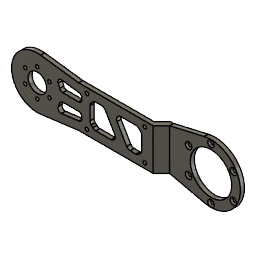
maker arm cnc装配 (Autodesk Fusion 360 archive; units mm, degrees)
design "L2输出侧臂"
part number: 2026-08-07-18-40-20-712
Autodesk Fusion 360 part; units mm, degrees
note: some values were not read from the file. Set by a fixed rule: the direction of a hole.
(part 1 of 4)
sketch "草图1" plane through (0, 0, 0) normal (0, 0, 1) x (1, 0, 0)
  line L0 (0, -20) -> (160, -20)
  arc A0 (160, -20) -> (160, 20) centre (160, 0) ccw
  line L1 (160, 20) -> (0, 20)
  arc A1 (0, 20) -> (0, -20) centre (0, 0) ccw
  line L2 (0, 0) -> (160, 0) construction
  line L3 (-10.3229, -9.3593) -> (-6.3955, -5.4319)
  arc A2 (-2.9439, 13.6195) -> (-5.8655, 15.1009) centre (-5.0689, 13.0501) ccw
  circle A3 centre (0, -13.5) radius 1.6
  arc A4 (16.0105, 2.4708) -> (13.2668, 4.2603) centre (13.8362, 2.1352) ccw
  circle A5 centre (-11.6913, 6.75) radius 1.6
  arc A6 (-5.8655, 15.1009) -> (-10.145, 12.6301) centre (0, 0) ccw
  line L4 (-1.5064, -8.2546) -> (-2.9439, -13.6195)
  circle A7 centre (-11.6913, -6.75) radius 1.6
  line L5 (7.9019, 2.8227) -> (13.2668, 4.2603)
  arc A8 (-2.6915, 5.6961) -> (-1.5064, 8.2547) centre (-3.6314, 7.6852) ccw
  circle A9 centre (6.115, -10.5915) radius 1.7
  circle A10 centre (6.115, 10.5915) radius 1.7
  circle A11 centre (11.6913, -6.75) radius 1.6
  circle A12 centre (11.6913, 6.75) radius 1.6
  arc A13 (-10.145, 12.6301) -> (-10.3229, 9.3593) centre (-8.7673, 10.9149) ccw
  arc A14 (-10.145, -12.6301) -> (-5.8655, -15.1009) centre (0, 0) ccw
  arc A15 (-2.6915, 5.6961) -> (-3.5872, 5.179) centre (0, 0) ccw
  arc A16 (13.2668, -4.2603) -> (16.0105, -2.4708) centre (13.8362, -2.1352) ccw
  arc A17 (6.2787, -0.5171) -> (7.9019, -2.8228) centre (8.4713, -0.6977) ccw
  circle A18 centre (0, 0) radius 18
  arc A19 (-1.5064, -8.2546) -> (-2.6915, -5.6961) centre (-3.6314, -7.6852) ccw
  circle A20 centre (-12.23, 0) radius 1.7
  line L6 (-6.3955, 5.4319) -> (-10.3229, 9.3593)
  circle A21 centre (0, 13.5) radius 1.6
  arc A22 (7.9019, 2.8227) -> (6.2787, 0.5171) centre (8.4713, 0.6977) ccw
  line L7 (-2.9439, 13.6195) -> (-1.5064, 8.2547)
  arc A23 (-5.8655, -15.1009) -> (-2.9439, -13.6195) centre (-5.0689, -13.0501) ccw
  arc A24 (6.2787, -0.5171) -> (6.2787, 0.5171) centre (0, 0) ccw
  arc A25 (-10.3229, -9.3593) -> (-10.145, -12.6301) centre (-8.7673, -10.9149) ccw
  arc A26 (16.0105, -2.4708) -> (16.0105, 2.4708) centre (0, 0) ccw
  arc A27 (-6.3955, 5.4319) -> (-3.5872, 5.179) centre (-4.8399, 6.9875) ccw
  line L8 (13.2668, -4.2603) -> (7.9019, -2.8228)
  circle A28 centre (0, 0) radius 4.75
  arc A29 (-3.5872, -5.179) -> (-2.6915, -5.6961) centre (0, 0) ccw
  arc A30 (-3.5872, -5.179) -> (-6.3955, -5.4319) centre (-4.8399, -6.9875) ccw
  circle A31 centre (160, 0) radius 28.5
  line L9 (153.5772, 27.7668) -> (120, 20)
  line L10 (120, -20) -> (153.5772, -27.7668)
  circle A32 centre (160, 0) radius 20
  circle A33 centre (160, 0) radius 25 construction
  circle A34 centre (160, 25) radius 1.65
  circle A35 centre (138.3494, 12.5) radius 1.65
  circle A36 centre (138.3494, -12.5) radius 1.65
  circle A37 centre (160, -25) radius 1.65
  circle A38 centre (181.6506, -12.5) radius 1.65
  circle A39 centre (181.6506, 12.5) radius 1.65
  circle A40 centre (0, 0) radius 25
  line L11 (3.2298, 24.7905) -> (40, 20)
  line L12 (3.2298, -24.7905) -> (40, -20)
  line L13 (160, 0) -> (160, 50)
  line L14 (160, 0) -> (160, 25)
  point P0 (0, 0)
  dimension "d1" = 20
  dimension "d2" = 160
  dimension "d3" = 36
  dimension "d4" = 3.2
  dimension "d5" = 57
  dimension "d6" = 40
  dimension "d7" = 40
  dimension "d8" = 40
  dimension "d9" = 50
  dimension "d10" = 3.3
  dimension "d12" = 360
  dimension "d15" = 50
  dimension "d92" = 40
  constraint tangent L0 A0
  constraint tangent A0 L1
  constraint parallel L0 L1
  constraint tangent L1 A1
  constraint tangent L0 A1
  constraint horizontal L2
  constraint coincident A1.centre L2.start
  constraint equal A12 A21
  constraint equal A11 A12
  constraint equal A3 A11
  constraint equal A3 A7
  constraint equal A5 A7
  constraint concentric A0 A31
  constraint coincident A31 L9.start
  constraint coincident L1 L9.end
  constraint coincident L0 L10.start
  constraint coincident A31 L10.end
  constraint tangent A31 L9
  constraint tangent A31 L10
  constraint concentric A0 A32
  constraint concentric A31 A33
  constraint coincident A33 A34.centre
  constraint coincident P0 A1.centre
  constraint coincident A40 L11.start
  constraint coincident L1 L11.end
  constraint coincident A40 L12.start
  constraint coincident L0 L12.end
  constraint tangent A40 L11
  constraint tangent A40 L12
  constraint equal L11 L12
  constraint coincident A0.centre L2.end
  constraint perpendicular L2 L13
  constraint coincident A34.centre L14.end
  constraint vertical L14
  measures "d1" radius of A1
  measures "d2" distance of P0 A0.centre
  measures "d3" diameter of A18
  measures "d4" diameter of A21
  measures "d5" diameter of A31
  measures "d6" horizontal distance of A0.centre L9.end
  measures "d7" horizontal distance of A0.centre L10.start
  measures "d8" diameter of A32
  measures "d9" diameter of A33
  measures "d10" diameter of A34
  measures "d15" diameter of A40
  measures "d92" horizontal distance of P0 L11.end
extrude "拉伸1" add sketch "草图1" along normal blind 4 contours L0 L1 A31 A40 | L0 A40 L12 | L0 A31 L10 | L0 L1 A1 A40 | L0 L1 A1 A40 | L0 L1 A31 A32 | L0 A0 A31 A32 A34 L13 L14 | L1 A40 L11 | L1 A31 A34 L13 L14 | L1 A31 L9 | L3 L4 A14 A19 A23 A25 A29 A30 | A2 A6 A8 A13 A15 L6 L7 A27 | A4 L5 A16 A17 A22 A24 A26 L8 | A9 | A10 | A18 | A20
sketch "草图3" plane through (0, 0, 4) normal (0, 0, 1) x (1, 0, 0)
  circle A0 centre (160, -25) radius 1.65
  circle A1 centre (181.6506, -12.5) radius 1.65
  circle A2 centre (181.6506, 12.5) radius 1.65
  arc A3 (3.2298, 24.7905) -> (3.2298, -24.7905) centre (0, 0) ccw
  line L0 (3.2298, -24.7905) -> (40, -20)
  line L1 (40, -20) -> (120, -20)
  line L2 (120, -20) -> (153.5772, -27.7668)
  arc A4 (153.5772, -27.7668) -> (153.5772, 27.7668) centre (160, 0) ccw
  line L3 (153.5772, 27.7668) -> (120, 20)
  line L4 (120, 20) -> (40, 20)
  line L5 (40, 20) -> (3.2298, 24.7905)
  circle A5 centre (0, -13.5) radius 1.6
  circle A6 centre (160, 25) radius 1.65
  circle A7 centre (-11.6913, 6.75) radius 1.6
  circle A8 centre (11.6913, 6.75) radius 1.6
  circle A9 centre (11.6913, -6.75) radius 1.6
  circle A10 centre (-11.6913, -6.75) radius 1.6
  circle A11 centre (138.3494, 12.5) radius 1.65
  circle A12 centre (0, 0) radius 4.75
  circle A13 centre (138.3494, -12.5) radius 1.65
  circle A14 centre (0, 13.5) radius 1.6
  circle A15 centre (160, 0) radius 20
  arc A16 (0, 24.5) -> (-21.2176, 12.25) centre (0, 0) ccw
  arc A17 (0, 19.5) -> (0, 24.5) centre (0, 22) ccw
  arc A18 (0, 19.5) -> (-16.8875, 9.75) centre (0, 0) ccw
  arc A19 (-21.2176, 12.25) -> (-16.8875, 9.75) centre (-19.0526, 11) ccw
  arc A20 (0, 22) -> (-19.0526, 11) centre (0, 0) ccw construction
  line L6 (-19.0526, 11) -> (0, 0)
  line L7 (0, 0) -> (0, 22)
  line L8 (0, 0) -> (0, 80)
  arc A21 (-21.2176, -12.25) -> (0, -24.5) centre (0, 0) ccw
  arc A22 (-16.8875, -9.75) -> (-21.2176, -12.25) centre (-19.0526, -11) ccw
  arc A23 (-16.8875, -9.75) -> (0, -19.5) centre (0, 0) ccw
  arc A24 (0, -24.5) -> (0, -19.5) centre (0, -22) ccw
  arc A25 (21.2176, -12.25) -> (21.2176, 12.25) centre (0, 0) ccw
  arc A26 (16.8875, -9.75) -> (21.2176, -12.25) centre (19.0526, -11) ccw
  arc A27 (16.8875, -9.75) -> (16.8875, 9.75) centre (0, 0) ccw
  arc A28 (21.2176, 12.25) -> (16.8875, 9.75) centre (19.0526, 11) ccw
  dimension "d19" = 5
  dimension "d20" = 22
  dimension "d22" = 60
  dimension "d24" = 360
  constraint tangent A16 A17
  constraint tangent A17 A18
  constraint tangent A18 A19
  constraint tangent A16 A19
  constraint coincident A3.centre A12.centre
  constraint coincident A19.centre A20.end
  constraint coincident A17.centre A20.start
  constraint vertical L8
  constraint coincident A17.centre L8
  measures "d19" diameter of A19
  measures "d20" radius of A20
  measures "d22" angle of L6 L7
extrude "拉伸4" add 1 faces at (66.6667, 6.6667, 4) along direction (0, 0, 1) blind 8
sketch "草图5" plane through (0, -20, 0) normal (0, -1, 0) x (1, 0, 0)
  line L0 (40, 0) -> (120, 0)
  line L1 (120, 0) -> (120, 12)
  line L2 (120, 12) -> (40, 12)
  line L3 (40, 12) -> (40, 0)
  line L4 (3.2298, 0) -> (-25, 0)
  line L5 (3.2298, 0) -> (3.2298, 12)
  line L6 (3.2298, 12) -> (-25, 12)
  line L7 (3.2298, 12) -> (3.2298, 0)
  line L8 (-25, 12) -> (-25, 0)
  line L9 (-29.5, 8) -> (40, 8)
  line L10 (40, 8) -> (40, 0)
  line L11 (40, 0) -> (-29.5, 0)
  line L12 (-29.5, 0) -> (-29.5, 8)
  line L13 (120, 12) -> (197.6265, 12)
  line L14 (197.6265, 12) -> (197.6265, 4)
  line L15 (197.6265, 4) -> (120, 4)
  line L16 (120, 4) -> (120, 12)
  dimension "d41" = 8
  dimension "d42" = 8
  constraint coincident L6.end L8.start
  constraint coincident L4.end L8.end
  constraint horizontal L9
  constraint vertical L10
  constraint horizontal L11
  constraint vertical L12
  constraint coincident L0.start L3.end
  constraint horizontal L13
  constraint vertical L14
  constraint horizontal L15
  constraint vertical L16
  constraint coincident L1.end L2.start
  measures "d41" distance of L9.end L0.start
  measures "d42" distance of L13.end L14.end
extrude "拉伸5" cut sketch "草图5" along normal blind -120 and the other way blind -45 contours L3 L5 L7 L9 L10 L11 | L4 L5 L7 L8 L9 L11 | L1 L13 L14 L15 L16 | L8 L9 L11 L12
sketch "草图6" plane through (0, -20, 0) normal (0, -1, 0) x (1, 0, 0)
  line L0 (120, 12) -> (40, 12)
  line L1 (40, 12) -> (40, 8)
  line L2 (40, 0) -> (116.9289, 0)
  line L3 (120, 0) -> (120, 4)
  line L4 (40, 8) -> (108.9289, 8)
  line L5 (108.9289, 8) -> (108.9289, 0)
  line L6 (108.9289, 0) -> (40, 0)
  line L7 (40, 0) -> (40, 8)
  line L8 (108.9289, 8) -> (116.9289, 0)
  line L9 (120, 4) -> (120, 12)
  line L10 (40, 8) -> (40, 0)
  line L11 (112, 12) -> (120, 4)
  line L12 (116.9289, 0) -> (108.9289, 0)
  dimension "d60" = 45
  dimension "d61" = 5
  constraint horizontal L4
  constraint vertical L5
  constraint horizontal L6
  constraint vertical L7
  constraint coincident L2 L5.end
  constraint coincident L1.end L4.start
  constraint coincident L0 L11.start
  constraint coincident L3.end L9.start
  constraint parallel L8 L11
  measures "d60" angle of L0 L11
  measures "d61" distance of L8 L11
extrude "拉伸6" cut sketch "草图6" against normal blind 69
sketch "草图7" plane through (0, 0, 12) normal (0, 0, 1) x (1, 0, 0)
  line L0 (112, -20) -> (112, 20)
  line L1 (112, 20) -> (40, 20)
  line L2 (40, 20) -> (3.2298, 24.7905)
  arc A0 (3.2298, 24.7905) -> (3.2298, -24.7905) centre (0, 0) ccw
  line L3 (3.2298, -24.7905) -> (40, -20)
  line L4 (40, -20) -> (112, -20)
  circle A1 centre (-11.6913, 6.75) radius 1.6
  circle A2 centre (-11.6913, -6.75) radius 1.6
  circle A3 centre (11.6913, -6.75) radius 1.6
  circle A4 centre (0, 13.5) radius 1.6
  circle A5 centre (0, -13.5) radius 1.6
  circle A6 centre (0, 0) radius 4.75
  circle A7 centre (11.6913, 6.75) radius 1.6
  line L5 (48, 15) -> (104, 15) construction
  line L6 (104, 15) -> (104, -15) construction
  line L7 (104, -15) -> (48, -15) construction
  line L8 (48, -15) -> (48, 15) construction
  circle A8 centre (48, 15) radius 1.65
  circle A9 centre (104, 15) radius 1.65
  circle A10 centre (48, -15) radius 1.65
  circle A11 centre (104, -15) radius 1.65
  line L9 (51, -8.1005) -> (51, 8.1005)
  line L10 (101, 8.1005) -> (101, -8.1005)
  line L11 (51, 8.1005) -> (54.8995, 12)
  line L12 (97.1005, 12) -> (101, 8.1005)
  line L13 (54.8995, -12) -> (51, -8.1005)
  line L14 (97.1005, -12) -> (101, -8.1005)
  line L15 (64.453, 12) -> (78.3094, -12)
  line L16 (87.547, -12) -> (73.6906, 12)
  line L17 (54.8995, 12) -> (64.453, 12)
  line L18 (73.6906, 12) -> (97.1005, 12)
  line L19 (97.1005, -12) -> (87.547, -12)
  line L20 (78.3094, -12) -> (54.8995, -12)
  point P0 (101, -12)
  point P1 (51, -12)
  point P2 (51, 12)
  point P3 (101, 12)
  dimension "d62" = 5
  dimension "d63" = 8
  dimension "d64" = 5
  dimension "d65" = 8
  dimension "d79" = 7
  dimension "d80" = 45
  dimension "d82" = 135
  dimension "d83" = 45
  dimension "d84" = 135
  dimension "d86" = 60
  dimension "d87" = 8
  dimension "d100" = 3.3
  constraint horizontal L5
  constraint vertical L6
  constraint horizontal L7
  constraint vertical L8
  constraint coincident L5.start L8.end
  constraint coincident L5.end L6.start
  constraint coincident L7.end L8.start
  constraint coincident L6.end L7.start
  constraint equal A8 A9
  constraint equal A8 A10
  constraint equal A8 A11
  constraint coincident P2 L9
  constraint coincident P2 L17
  constraint coincident P3 L18
  constraint coincident P3 L10
  constraint coincident P1 L20
  constraint coincident P1 L9
  constraint coincident P0 L19
  constraint coincident P0 L10
  constraint equal L11 L12
  constraint equal L12 L13
  constraint equal L12 L14
  constraint parallel L15 L16
  constraint collinear L17 L18
  constraint collinear L19 L20
  constraint equal L17 L19
  measures "d62" distance of L1 L5
  measures "d63" distance of L0 L6
  measures "d64" distance of L4 L7
  measures "d65" distance of L1.end L8
  measures "d79" distance of L5.start L11
  measures "d80" angle of L11 L17
  measures "d82" angle of L12 L18
  measures "d83" angle of L13 L20
  measures "d84" angle of L14 L19
  measures "d86" angle of L15 L20
  measures "d87" distance of L15 L16
  measures "d100" diameter of A8
extrude "拉伸7" cut sketch "草图7" against normal blind 75 contours A8 | A9 | A10 | A11
extrude "拉伸8" cut sketch "草图7" against normal blind 27 contours L9 L11 L13 L15 L17 L20 | L10 L12 L14 L16 L18 L19
fillet "圆角4" radius 4 12 edges at (54.8995, -12, 10) (51, -8.1005, 10) (51, 8.1005, 10) (54.8995, 12, 10) (64.453, 12, 10) (78.3094, -12, 10) (73.6906, 12, 10) (87.547, -12, 10) (97.1005, -12, 10) (101, -8.1005, 10) (101, 8.1005, 10) (97.1005, 12, 10)
sketch "草图8" plane through (0, 0, 8) normal (0, 0, 1) x (1, 0, 0)
  circle A0 centre (104, 15) radius 3.15
  circle A1 centre (104, 15) radius 1.65
  circle A2 centre (104, -15) radius 1.65
  circle A3 centre (48, 15) radius 1.65
  circle A4 centre (48, -15) radius 1.65
  circle A5 centre (48, 15) radius 3.15
  circle A6 centre (104, -15) radius 3.15
  circle A7 centre (48, -15) radius 3.15
  dimension "d120" = 6.3
  constraint concentric A3 A5
  constraint concentric A2 A6
  constraint concentric A4 A7
  constraint equal A0 A5
  constraint equal A5 A6
  constraint equal A5 A7
  constraint coincident A0.centre A1.centre
  measures "d120" diameter of A0
extrude "拉伸9" cut sketch "草图8" along normal blind 1.5
sketch "草图9" plane through (0, 0, 12) normal (0, 0, 1) x (1, 0, 0)
  circle A0 centre (104, 15) radius 1.65
  circle A1 centre (48, -15) radius 1.65
  circle A2 centre (48, 15) radius 1.65
  circle A3 centre (104, -15) radius 1.65
  circle A4 centre (11.6913, 6.75) radius 1.6
  circle A5 centre (0, 13.5) radius 1.6
  circle A6 centre (11.6913, -6.75) radius 1.6
  circle A7 centre (0, 0) radius 4.75
  circle A8 centre (-11.6913, -6.75) radius 1.6
  circle A9 centre (0, -13.5) radius 1.6
  circle A10 centre (-11.6913, 6.75) radius 1.6
  line L0 (112, -20) -> (112, 20)
  line L1 (112, 20) -> (40, 20)
  line L2 (40, 20) -> (3.2298, 24.7905)
  arc A11 (3.2298, 24.7905) -> (3.2298, -24.7905) centre (0, 0) ccw
  line L3 (3.2298, -24.7905) -> (40, -20)
  line L4 (40, -20) -> (112, -20)
  line L5 (101, 6.4437) -> (101, -6.4437)
  arc A12 (99.8284, -9.2721) -> (101, -6.4437) centre (97, -6.4437) ccw
  line L6 (99.8284, -9.2721) -> (98.2721, -10.8284)
  arc A13 (95.4437, -12) -> (98.2721, -10.8284) centre (95.4437, -8) ccw
  line L7 (95.4437, -12) -> (89.8564, -12)
  arc A14 (86.3923, -10) -> (89.8564, -12) centre (89.8564, -8) ccw
  line L8 (86.3923, -10) -> (77.1547, 6)
  arc A15 (80.6188, 12) -> (77.1547, 6) centre (80.6188, 8) ccw
  line L9 (80.6188, 12) -> (95.4437, 12)
  arc A16 (98.2721, 10.8284) -> (95.4437, 12) centre (95.4437, 8) ccw
  line L10 (98.2721, 10.8284) -> (99.8284, 9.2721)
  arc A17 (101, 6.4437) -> (99.8284, 9.2721) centre (97, 6.4437) ccw
  line L11 (56.5563, 12) -> (62.1436, 12)
  arc A18 (65.6077, 10) -> (62.1436, 12) centre (62.1436, 8) ccw
  line L12 (65.6077, 10) -> (74.8453, -6)
  arc A19 (71.3812, -12) -> (74.8453, -6) centre (71.3812, -8) ccw
  line L13 (71.3812, -12) -> (56.5563, -12)
  arc A20 (53.7279, -10.8284) -> (56.5563, -12) centre (56.5563, -8) ccw
  line L14 (53.7279, -10.8284) -> (52.1716, -9.2721)
  arc A21 (51, -6.4437) -> (52.1716, -9.2721) centre (55, -6.4437) ccw
  line L15 (51, -6.4437) -> (51, 6.4437)
  arc A22 (52.1716, 9.2721) -> (51, 6.4437) centre (55, 6.4437) ccw
  line L16 (52.1716, 9.2721) -> (53.7279, 10.8284)
  arc A23 (56.5563, 12) -> (53.7279, 10.8284) centre (56.5563, 8) ccw
  circle A24 centre (0, 0) radius 9
  dimension "d97" = 18
  constraint concentric A7 A24
  measures "d97" diameter of A24
extrude "拉伸10" cut sketch "草图9" against normal blind 9 contours A24
sketch "草图11" plane through (0, 0, 12) normal (0, 0, 1) x (1, 0, 0)
  arc A0 (16.8121, -14.9533) -> (16.8121, 14.9533) centre (0, 0) ccw
  line L0 (16.8121, 14.9533) -> (43, 11.5415)
  line L1 (43, 11.5415) -> (43, -11.5415)
  line L2 (43, -11.5415) -> (16.8121, -14.9533)
  line L3 (0, 0) -> (43, 0) construction
  line L4 (22.1416, 4) -> (43, 4)
  line L5 (22.1416, -4) -> (43, -4)
  line L6 (40, 20) -> (3.2298, 24.7905)
  line L7 (51, -6.4437) -> (51, 6.4437)
  dimension "d112" = 8
  dimension "d113" = 22.5
  dimension "d114" = 8
  dimension "d117" = 8
  constraint coincident A0.centre L3.start
  constraint vertical L1
  constraint midpoint L1 L3.end
  constraint horizontal L3
  constraint symmetric A0.start A0.end L3
  constraint coincident A0 L4.start
  constraint coincident L1 L4.end
  constraint perpendicular L1 L4
  constraint coincident A0 L5.start
  constraint coincident L1 L5.end
  constraint perpendicular L1 L5
  constraint symmetric L3 L4.start L5.start
  constraint parallel L0 L6
  measures "d112" distance of L0 L6
  measures "d113" radius of A0
  measures "d114" distance of L4 L5
  measures "d117" distance of L1 L7
extrude "拉伸11" cut sketch "草图11" against normal blind 26 contours A0 L1 L2 L5 | A0 L0 L1 L4
fillet "圆角5" radius 3 8 edges at (16.8121, 14.9533, 10) (43, 11.5415, 10) (43, 4, 10) (22.1416, 4, 10) (16.8121, -14.9533, 10) (22.1416, -4, 10) (43, -4, 10) (43, -11.5415, 10)
sketch "草图12" plane through (0, 0, 4) normal (0, 0, 1) x (1, 0, 0)
  circle A0 centre (181.6506, -12.5) radius 1.65
  circle A1 centre (160, -25) radius 1.65
  circle A2 centre (181.6506, 12.5) radius 1.65
  circle A3 centre (160, 0) radius 20
  circle A4 centre (160, 25) radius 1.65
  circle A5 centre (138.3494, 12.5) radius 1.65
  circle A6 centre (138.3494, -12.5) radius 1.65
  line L0 (120, -20) -> (153.5772, -27.7668)
  arc A7 (153.5772, -27.7668) -> (153.5772, 27.7668) centre (160, 0) ccw
  line L1 (153.5772, 27.7668) -> (120, 20)
  line L2 (120, 20) -> (120, -20)
hole "孔1" at (160, -25, 4) at (138.3494, -12.5, 4) at (181.6506, -12.5, 4) at (181.6506, 12.5, 4) at (138.3494, 12.5, 4) at (160, 25, 4) direction (0, 0, -1) diameter 3.3 depth 8 tip angle 180 countersink diameter 6.3 countersink angle 90

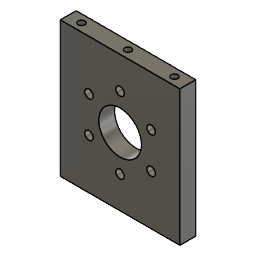
design "L2电机固定底板"
part number: 2026-08-07-13-29-31-729
Autodesk Fusion 360 part; units mm, degrees
sketch "草图1" plane through (0, 0, 0) normal (0, 0, 1) x (1, 0, 0)
  line L0 (22.5, 25.5) -> (-22.5, 25.5)
  line L1 (-22.5, 25.5) -> (-22.5, -25.5)
  line L2 (-22.5, -25.5) -> (22.5, -25.5)
  line L3 (22.5, -25.5) -> (22.5, 25.5)
  line L4 (22.5, 25.5) -> (-22.5, -25.5) construction
  line L5 (-22.5, 25.5) -> (22.5, -25.5) construction
  dimension "d1" = 51
  dimension "d2" = 45
  constraint horizontal L0
  constraint perpendicular L0 L1
  constraint parallel L0 L2
  constraint parallel L1 L3
  constraint coincident L4 origin
  constraint coincident L5 origin
  measures "d1" distance of L0.start L2.end
  measures "d2" distance of L0.start L0.end
extrude "拉伸1" add sketch "草图1" along normal blind 6
sketch "草图2" plane through (-22.5, 0, 0) normal (-1, 0, 0) x (0, 0, 1)
  line L0 (0, 25.5) -> (0, -25.5)
  line L1 (0, -25.5) -> (6, -25.5)
  line L2 (6, -25.5) -> (6, 25.5)
  line L3 (6, 25.5) -> (0, 25.5)
sketch "草图3" plane through (0, -25.5, 0) normal (0, -1, 0) x (1, 0, 0)
  line L0 (-22.5, 0) -> (22.5, 0)
  line L1 (22.5, 0) -> (22.5, 6)
  line L2 (22.5, 6) -> (-22.5, 6)
  line L3 (-22.5, 6) -> (-22.5, 0)
  circle A0 centre (17.5, 3) radius 1.25
  circle A1 centre (0, 3) radius 1.25
  circle A2 centre (-17.5, 3) radius 1.25
  dimension "d5" = 2.5
  dimension "d6" = 3
  dimension "d7" = 5
  dimension "d10" = 35
  dimension "d11" = 0
  measures "d5" diameter of A0
  measures "d6" distance of L2 A0.centre
  measures "d7" distance of L1 A0.centre
extrude "拉伸2" cut sketch "草图3" against normal blind 8 contours A0 | A1 | A2
mirror "镜像1" about plane through (0, 0, 0) normal (0, 1, 0) of "拉伸2"
sketch "草图4" plane through (0, 0, 0) normal (0, 0, -1) x (-1, 0, 0)
  line L0 (-22.5, 25.5) -> (-22.5, -25.5)
  line L1 (-22.5, -25.5) -> (22.5, -25.5)
  line L2 (22.5, -25.5) -> (22.5, 25.5)
  line L3 (22.5, 25.5) -> (-22.5, 25.5)
  circle A0 centre (0, 0) radius 13.5 construction
  circle A1 centre (0, 13.5) radius 1.6
  circle A2 centre (-11.6913, 6.75) radius 1.6
  circle A3 centre (-11.6913, -6.75) radius 1.6
  circle A4 centre (0, -13.5) radius 1.6
  circle A5 centre (11.6913, -6.75) radius 1.6
  circle A6 centre (11.6913, 6.75) radius 1.6
  circle A7 centre (0, 0) radius 8
  dimension "d16" = 27
  dimension "d17" = 3.2
  dimension "d19" = 360
  dimension "d20" = 16
  constraint coincident A0.centre A7.centre
  constraint coincident A0 A1.centre
  constraint vertical A1.centre A4.centre
  measures "d16" diameter of A0
  measures "d17" diameter of A1
  measures "d20" diameter of A7
extrude "拉伸3" cut sketch "草图4" against normal blind 41 contours A1 | A2 | A3 | A4 | A5 | A6 | A7
sketch "草图5" plane through (0, 0, 0) normal (0, 0, -1) x (-1, 0, 0)
  line L0 (-22.5, 25.5) -> (-22.5, -25.5)
  line L1 (-22.5, -25.5) -> (22.5, -25.5)
  line L2 (22.5, -25.5) -> (22.5, 25.5)
  line L3 (22.5, 25.5) -> (-22.5, 25.5)
  circle A0 centre (0, 0) radius 8
  circle A1 centre (-11.6913, -6.75) radius 1.6
  circle A2 centre (-11.6913, 6.75) radius 1.6
  circle A3 centre (11.6913, -6.75) radius 1.6
  circle A4 centre (0, -13.5) radius 1.6
  circle A5 centre (0, 13.5) radius 1.6
  circle A6 centre (11.6913, 6.75) radius 1.6
  circle A7 centre (0, 13.5) radius 3
  circle A8 centre (-11.6913, 6.75) radius 3
  circle A9 centre (-11.6913, -6.75) radius 3
  circle A10 centre (0, -13.5) radius 3
  circle A11 centre (11.6913, -6.75) radius 3
  circle A12 centre (11.6913, 6.75) radius 3
  dimension "d23" = 6
  dimension "d25" = 360
  constraint concentric A5 A7
  measures "d23" diameter of A7
extrude "拉伸4" cut sketch "草图5" against normal blind 3 contours A7 | A8 | A9 | A10 | A11 | A12

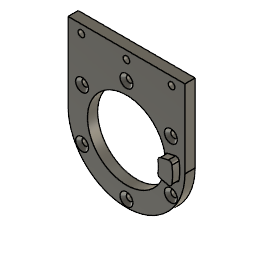
design "J5-J6-Out"
part number: 2026-08-07-16-54-43-717
Autodesk Fusion 360 part; units mm, degrees
sketch "草图1" plane through (0, 0, 0) normal (0, 1, 0) x (1, 0, 0)
  arc A0 (28.5, 0) -> (-28.5, 0) centre (0, 0) ccw
  line L0 (-28.5, 0) -> (-28.5, -38)
  line L1 (-28.5, -38) -> (28.5, -38)
  line L2 (28.5, -38) -> (28.5, 0)
  circle A1 centre (0, 0) radius 19
  circle A2 centre (0, 0) radius 25 construction
  circle A3 centre (-21.6506, -12.5) radius 1.6
  circle A4 centre (0, -25) radius 1.6
  circle A5 centre (21.6506, -12.5) radius 1.6
  circle A6 centre (21.6506, 12.5) radius 1.6
  circle A7 centre (0, 25) radius 1.6
  circle A8 centre (-21.6506, 12.5) radius 1.6
  circle A9 centre (22, -34) radius 1.6
  circle A10 centre (-22, -34) radius 1.6
  line L3 (0, 0) -> (0, -38) construction
  circle A11 centre (0, -34) radius 1.6
  line L4 (22, -34) -> (-22, -34) construction
  dimension "d1" = 28.5
  dimension "d2" = 50
  dimension "d3" = 38
  dimension "d4" = 3.2
  dimension "d6" = 360
  dimension "d7" = 38
  dimension "d10" = 3.2
  dimension "d11" = 44
  dimension "d12" = 4
  constraint coincident A0.centre A1.centre
  constraint tangent A0 L0
  constraint vertical L0
  constraint perpendicular L0 L1
  constraint perpendicular L1 L2
  constraint concentric A1 A2
  constraint coincident A2 A3.centre
  constraint tangent A0 L2
  constraint midpoint L1 L3.end
  constraint equal A9 A10
  constraint symmetric A9.centre A10.centre L3
  constraint coincident L3 A11.centre
  constraint equal A10 A11
  constraint coincident A9.centre L4.start
  constraint coincident A10.centre L4.end
  constraint midpoint A11.centre L4
  constraint coincident A4.centre L3
  measures "d1" radius of A0
  measures "d2" diameter of A2
  measures "d3" diameter of A1
  measures "d4" diameter of A3
  measures "d7" distance of L1 A0.centre
  measures "d10" diameter of A9
  measures "d11" distance of A9.centre A10.centre
  measures "d12" distance of L1 L4
extrude "拉伸1" add sketch "草图1" along normal blind 5
sketch "草图2" plane through (0, 0, 0) normal (0, -1, 0) x (1, 0, 0)
  circle A0 centre (0, 0) radius 19
  line L0 (28.5, 0) -> (28.5, 38)
  line L1 (28.5, 38) -> (-28.5, 38)
  line L2 (-28.5, 38) -> (-28.5, 0)
  arc A1 (-28.5, 0) -> (28.5, 0) centre (0, 0) ccw
  circle A2 centre (-22, 34) radius 1.6
  circle A3 centre (0, 34) radius 1.6
  circle A4 centre (-21.6506, -12.5) radius 1.6
  circle A5 centre (0, 25) radius 1.6
  circle A6 centre (21.6506, 12.5) radius 1.6
  circle A7 centre (21.6506, -12.5) radius 1.6
  circle A8 centre (-21.6506, 12.5) radius 1.6
  circle A9 centre (0, -25) radius 1.6
  circle A10 centre (22, 34) radius 1.6
  arc A11 (18.5496, -4.1124) -> (18.5496, 4.1124) centre (0, 0) ccw
  arc A12 (25.3837, -5.6274) -> (25.3837, 5.6274) centre (0, 0) ccw
  line L3 (0, 0) -> (26, 0) construction
  line L4 (25.3837, 5.6274) -> (18.5496, 4.1124)
  line L5 (18.5496, -4.1124) -> (25.3837, -5.6274)
  dimension "d13" = 19
  dimension "d14" = 25
  dimension "d15" = 26
  constraint coincident A0.centre A1.centre
  constraint midpoint A12 L3.end
  constraint coincident A0.centre L4
  constraint coincident A0.centre L5
  constraint horizontal L3
  measures "d13" radius of A11
  measures "d14" angle of L4 L5
  measures "d15" radius of A12
extrude "拉伸2" add sketch "草图2" along normal blind 3.5 contours A0 A11 A12 L4 L5
fillet "圆角1" radius 1.5 4 edges at (25.3837, -1.75, 5.6274) (18.5496, -1.75, 4.1124) (25.3837, -1.75, -5.6274) (18.5496, -1.75, -4.1124)
hole "孔1" at (0, 0, 25) at (21.6506, 0, 12.5) at (21.6506, 0, -12.5) at (0, 0, -25) at (-21.6506, 0, -12.5) at (-21.6506, 0, 12.5) direction (0, 1, 0) diameter 3.2 depth 10 tip angle 180 countersink diameter 6.3 countersink angle 90
equation "d1 = ( 57 / 2 ) * 1 mm"

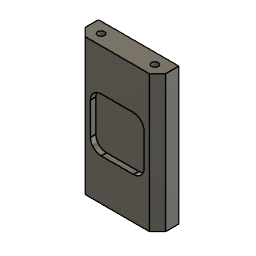
design "电机支撑"
part number: 2026-08-10-18-43-27-158
Autodesk Fusion 360 part; units mm, degrees
sketch "草图1" plane through (0, 0, 0) normal (0, 1, 0) x (1, 0, 0)
  line L0 (0, 0) -> (30, 0)
  line L1 (30, 0) -> (30, 8)
  line L2 (30, 8) -> (0, 8)
  line L3 (0, 8) -> (0, 0)
  circle A0 centre (5, 4) radius 1.25
  circle A1 centre (25, 4) radius 1.25
  dimension "d1" = 8
  dimension "d2" = 4
  dimension "d3" = 2.5
  dimension "d4" = 30
  dimension "d5" = 5
  dimension "d8" = 20
  dimension "d9" = 0
  constraint horizontal L0
  constraint vertical L1
  constraint horizontal L2
  constraint vertical L3
  constraint coincident L0.start L3.end
  measures "d1" distance of L0.start L2.end
  measures "d2" distance of L0 A0.centre
  measures "d3" diameter of A0
  measures "d4" distance of L1.end L2.end
  measures "d5" distance of L3 A0.centre
extrude "拉伸1" add sketch "草图1" along normal blind 51 contours L0 L1 L2 L3 | A0 | A1
extrude "拉伸2" cut sketch "草图1" along normal blind 6 contours A0 | A1
chamfer "倒角1" distance 3 angle 45 2 edges at (30, 25.5, 0) (0, 25.5, 0)
ref_plane "工作平面1" through (15, 25.5, -4) normal (0, -1, 0) x (-1, 0, 0)
mirror "镜像1" about plane through (15, 25.5, -4) normal (0, -1, 0) of "拉伸2"
sketch "草图2" plane through (0, 0, 0) normal (0, 0, 1) x (1, 0, 0)
  line L0 (3, 51) -> (3, 0)
  line L1 (3, 0) -> (27, 0)
  line L2 (27, 0) -> (27, 51)
  line L3 (27, 51) -> (3, 51)
  line L4 (0, 0) -> (30, 0)
  line L5 (5, 35.5) -> (25, 35.5)
  line L6 (25, 35.5) -> (25, 15.5)
  line L7 (25, 15.5) -> (5, 15.5)
  line L8 (5, 15.5) -> (5, 35.5)
  dimension "d25" = 2
  dimension "d26" = 2
  dimension "d27" = 15.5
  dimension "d28" = 15.5
  constraint horizontal L5
  constraint vertical L6
  constraint horizontal L7
  constraint vertical L8
  measures "d25" distance of L0 L8
  measures "d26" distance of L2 L6
  measures "d27" distance of L3 L5
  measures "d28" distance of L4 L7
extrude "拉伸4" cut sketch "草图2" against normal blind 2 contours L5 L6 L7 L8
fillet "圆角2" radius 4 4 edges at (5, 35.5, -1) (25, 35.5, -1) (25, 15.5, -1) (5, 15.5, -1)

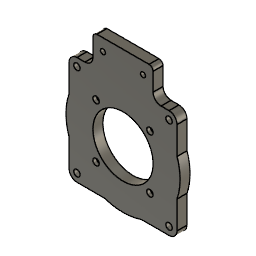
design "J7电机底座-平底"
part number: 2026-07-23-14-49-36-940
Autodesk Fusion 360 part; units mm, degrees
sketch "草图1" plane through (0, 0, 0) normal (0, 1, 0) x (1, 0, 0)
  circle A0 centre (0, 0) radius 28.5
  circle A1 centre (0, 0) radius 15
  circle A2 centre (0, 0) radius 19 construction
  line L0 (0, 0) -> (0, -28.5) construction
  circle A3 centre (-13.435, -13.435) radius 1.6
  circle A4 centre (13.435, -13.435) radius 1.6
  circle A5 centre (13.435, 13.435) radius 1.6
  circle A6 centre (-13.435, 13.435) radius 1.6
  circle A7 centre (-13.435, -13.435) radius 3
  circle A8 centre (13.435, -13.435) radius 3
  circle A9 centre (13.435, 13.435) radius 3
  circle A10 centre (-13.435, 13.435) radius 3
  circle A11 centre (0, 0) radius 32.5 construction
  line L1 (0, 0) -> (33, 0) construction
  circle A12 centre (22.981, -22.981) radius 1.6
  line L2 (9.1803, -26.981) -> (22.981, -26.981)
  arc A13 (22.981, -26.981) -> (26.981, -22.981) centre (22.981, -22.981) ccw
  line L3 (26.981, -22.981) -> (26.981, -9.1803)
  line L4 (26.981, 9.1803) -> (26.981, 22.981)
  arc A14 (26.981, 22.981) -> (22.981, 26.981) centre (22.981, 22.981) ccw
  line L5 (22.981, 26.981) -> (9.1803, 26.981)
  circle A15 centre (22.981, 22.981) radius 1.6
  line L6 (-9.1803, 26.981) -> (-22.981, 26.981)
  arc A16 (-22.981, 26.981) -> (-26.981, 22.981) centre (-22.981, 22.981) ccw
  line L7 (-26.981, 22.981) -> (-26.981, 9.1803)
  circle A17 centre (-22.981, 22.981) radius 1.6
  line L8 (-26.981, -9.1803) -> (-26.981, -22.981)
  arc A18 (-26.981, -22.981) -> (-22.981, -26.981) centre (-22.981, -22.981) ccw
  line L9 (-22.981, -26.981) -> (-9.1803, -26.981)
  circle A19 centre (-22.981, -22.981) radius 1.6
  dimension "d1" = 57
  dimension "d2" = 30
  dimension "d4" = 360
  dimension "d5" = 3.2
  dimension "d6" = 38
  dimension "d7" = 6
  dimension "d19" = 65
  dimension "d29" = 3.2
  dimension "d30" = 4
  dimension "d32" = 360
  constraint coincident A0.centre A1.centre
  constraint concentric A0 A1
  constraint coincident A0 L0.end
  constraint vertical L0
  constraint coincident A2 A3.centre
  constraint symmetric L0 A3.centre A4.centre
  constraint concentric A3 A7
  constraint concentric A0 A11
  constraint coincident A11 A12.centre
  constraint coincident A0 L2.start
  constraint horizontal L2
  constraint tangent L2 A13
  constraint coincident A0 L3.end
  constraint tangent A13 L3
  constraint coincident A12.centre A13.centre
  constraint vertical L3
  constraint symmetric L0 A12.centre A18.centre
  measures "d1" diameter of A0
  measures "d2" diameter of A1
  measures "d5" diameter of A3
  measures "d6" diameter of A2
  measures "d7" diameter of A7
  measures "d19" diameter of A11
  measures "d29" diameter of A12
  measures "d30" radius of A13
extrude "拉伸1" add sketch "草图1" along normal mid plane 5 contours A0 | A0 L4 A14 L5 | A0 L2 A13 L3 | A0 L6 A16 L7 | A0 L8 A18 L9 | A7 | A8 | A9 | A10
extrude "拉伸2" cut sketch "草图1" against normal blind 3.2 from surface at 2.5 contours A7 | A8 | A9 | A10
sketch "草图5" plane through (0, -2.5, 0) normal (0, -1, 0) x (1, 0, 0)
  circle A0 centre (-13.435, -13.435) radius 1.6
  circle A1 centre (13.435, 13.435) radius 1.6
  circle A2 centre (-22.981, 22.981) radius 1.6
  circle A3 centre (-22.981, -22.981) radius 1.6
  circle A4 centre (22.981, -22.981) radius 1.6
  circle A5 centre (-13.435, 13.435) radius 1.6
  circle A6 centre (13.435, -13.435) radius 1.6
  circle A7 centre (0, 0) radius 15
  line L0 (-9.1803, 26.981) -> (-22.981, 26.981)
  arc A8 (-22.981, 26.981) -> (-26.981, 22.981) centre (-22.981, 22.981) ccw
  line L1 (-26.981, 22.981) -> (-26.981, 9.1803)
  arc A9 (-26.981, 9.1803) -> (-26.981, -9.1803) centre (0, 0) ccw
  line L2 (-26.981, -9.1803) -> (-26.981, -22.981)
  arc A10 (-26.981, -22.981) -> (-22.981, -26.981) centre (-22.981, -22.981) ccw
  line L3 (-22.981, -26.981) -> (-9.1803, -26.981)
  arc A11 (-9.1803, -26.981) -> (9.1803, -26.981) centre (0, 0) ccw
  line L4 (9.1803, -26.981) -> (22.981, -26.981)
  arc A12 (22.981, -26.981) -> (26.981, -22.981) centre (22.981, -22.981) ccw
  line L5 (26.981, -22.981) -> (26.981, -9.1803)
  arc A13 (26.981, -9.1803) -> (26.981, 9.1803) centre (0, 0) ccw
  line L6 (26.981, 9.1803) -> (26.981, 22.981)
  arc A14 (26.981, 22.981) -> (22.981, 26.981) centre (22.981, 22.981) ccw
  line L7 (22.981, 26.981) -> (9.1803, 26.981)
  arc A15 (9.1803, 26.981) -> (-9.1803, 26.981) centre (0, 0) ccw
  circle A16 centre (22.981, 22.981) radius 1.6
  line L8 (-15, 26.981) -> (-15, 42)
  line L9 (-15, 42) -> (15, 42)
  line L10 (15, 42) -> (15, 26.981)
  line L11 (0, 0) -> (0, 42) construction
  circle A17 centre (-10, 36) radius 1.25
  circle A18 centre (10, 36) radius 1.25
  line L12 (-10, 36) -> (10, 36) construction
  dimension "d33" = 2.5
  dimension "d35" = 20
  dimension "d37" = 30
  dimension "d45" = 36
  dimension "d46" = 42
  constraint coincident L0 L8.start
  constraint parallel L0 L9
  constraint coincident L7 L10.end
  constraint coincident A7.centre A9.centre
  constraint midpoint L9 L11.end
  constraint vertical L11
  constraint symmetric L8.start L10.end L11
  constraint symmetric L11 A17.centre A18.centre
  constraint equal A17 A18
  constraint coincident A17.centre L12.start
  constraint coincident A18.centre L12.end
  constraint vertical L8
  measures "d33" diameter of A17
  measures "d35" distance of A17.centre A18.centre
  measures "d37" distance of L8.end L9.end
  measures "d45" distance of A7.centre L12
  measures "d46" distance of A7.centre L9
extrude "拉伸5" add sketch "草图5" against normal blind 5 contours L0 L7 A15 L8 L9 L10
fillet "圆角2" radius 4 2 edges at (-15, 0, 26.981) (15, 0, 26.981)
fillet "圆角2" radius 2 2 edges at (-15, 0, 42) (15, 0, 42)

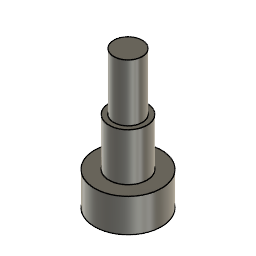
design "M4塞打螺栓"
part number: 2026-07-22-17-54-56-863
Autodesk Fusion 360 part; units mm, degrees
sketch "草图1" plane through (0, 0, 0) normal (0, 1, 0) x (1, 0, 0)
  line L0 (0, 0) -> (0, -14.5)
  line L1 (0, 0) -> (-3.5, 0)
  line L2 (-3.5, 0) -> (-3.5, -3.5)
  line L3 (-3.5, -3.5) -> (-2, -3.5)
  line L4 (-2, -3.5) -> (-2, -8.5)
  line L5 (-2, -8.5) -> (-1.5, -8.5)
  line L6 (-1.5, -8.5) -> (-1.5, -14.5)
  line L7 (-1.5, -14.5) -> (0, -14.5)
  line L8 (1.5, -14.5) -> (0, -14.5) construction
  line L9 (1.5, -8.5) -> (1.5, -14.5) construction
  line L10 (2, -8.5) -> (1.5, -8.5) construction
  line L11 (2, -3.5) -> (2, -8.5) construction
  line L12 (3.5, -3.5) -> (2, -3.5) construction
  line L13 (3.5, 0) -> (3.5, -3.5) construction
  line L14 (0, 0) -> (3.5, 0)
  dimension "d1" = 3
  dimension "d2" = 4
  dimension "d3" = 7
  dimension "d4" = 5
  dimension "d5" = 6
  dimension "d6" = 3.5
  constraint coincident L0.start L1.start
  constraint vertical L0
  constraint perpendicular L0 L1
  constraint perpendicular L1 L2
  constraint perpendicular L2 L3
  constraint perpendicular L3 L4
  constraint perpendicular L4 L5
  constraint perpendicular L5 L6
  constraint perpendicular L0 L7
  constraint symmetric L1.start L0 L14.start
  constraint symmetric L7.end L0 L8.end
  constraint symmetric L0 L1.end L13.start
  constraint symmetric L0 L2.end L12.start
  constraint symmetric L0 L3.end L11.start
  constraint symmetric L0 L4.end L10.start
  constraint symmetric L0 L5.end L9.start
  constraint symmetric L0 L6.end L8.start
  measures "d1" distance of L6 L9
  measures "d2" distance of L4 L11
  measures "d3" distance of L2 L13
  measures "d4" distance of L3.end L4.end
  measures "d5" distance of L5.end L6.end
  measures "d6" distance of L1.end L2.end
revolve "旋转1" add sketch "草图1" angle 360 about axis through (0, 0, 0) along (0, 0, 1)

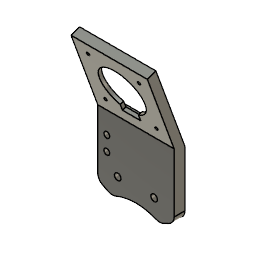
design "Maker Arm摄像头支架-2"
part number: 2026-08-07-11-14-49-423
Autodesk Fusion 360 part; units mm, degrees
sketch "草图2" plane through (0, 0, 0) normal (1, 0, 0) x (0, 1, 0)
  line L0 (-6, 64.7966) -> (-6, 0)
  line L1 (0, 62.9308) -> (0, 0)
  line L2 (-6, 0) -> (0, 0)
  line L3 (0, 62.9308) -> (-16.0084, 106.9135)
  line L4 (-16.0084, 106.9135) -> (-20.7069, 105.2034)
  line L5 (-20.7069, 105.2034) -> (-6, 64.7966)
  point P0 (-13.3534, 85)
  dimension "d70" = 6
  dimension "d71" = 5
  dimension "d72" = 43
  dimension "d73" = 160
  dimension "d74" = 85
  constraint vertical L0
  constraint vertical L1
  constraint perpendicular L1 L2
  constraint coincident L1.end L2.end
  constraint perpendicular L3 L4
  constraint perpendicular L4 L5
  constraint midpoint L5 P0
  measures "d70" distance of L0.end L1.end
  measures "d71" distance of L3.end L4.end
  measures "d72" distance of L0.start L4.end
  measures "d73" angle of L0 L5
  measures "d74" distance of L2 P0
extrude "拉伸2" add sketch "草图2" along normal mid plane 42
sketch "草图12" plane through (0, -6, 0) normal (0, -1, 0) x (1, 0, 0)
  line L0 (-21, 0) -> (21, 0)
  line L1 (21, 0) -> (21, 64.7966)
  line L2 (21, 64.7966) -> (-21, 64.7966)
  line L3 (-21, 64.7966) -> (-21, 0)
  circle A0 centre (0, 0) radius 28.5
  circle A1 centre (-10, 36) radius 1.8
  circle A2 centre (10, 36) radius 1.8
  line L4 (0, 0) -> (0, 28.5) construction
  dimension "d92" = 57
  dimension "d93" = 3.6
  dimension "d94" = 36
  dimension "d95" = 20
  constraint coincident A0.centre L4.start
  constraint coincident A0 L4.end
  constraint perpendicular L0 L4
  constraint symmetric A1.centre A2.centre L4
  constraint equal A1 A2
  measures "d92" diameter of A0
  measures "d93" diameter of A1
  measures "d94" vertical distance of A0.centre A1.centre
  measures "d95" distance of A1.centre A2.centre
extrude "拉伸13" cut sketch "草图12" against normal up to surface (6 mm away) contours L0 L1 L3 A0 | A1 | A2 picked at (0, 9.5)
sketch "草图10" plane through (0, 20.2256, 7.3615) normal (0, 0.939693, 0.34202) x (-1, 0, 0)
  line L0 (21, 105.941) -> (-21, 105.941)
  line L1 (-21, 105.941) -> (-21, 59.1356)
  line L2 (-21, 59.1356) -> (21, 59.1356)
  line L3 (21, 59.1356) -> (21, 105.941)
  line L4 (0, 105.941) -> (0, 59.1356) construction
  line L5 (-19.5, 65.441) -> (19.5, 65.441)
  line L6 (19.5, 65.441) -> (19.5, 104.441)
  line L7 (19.5, 104.441) -> (-19.5, 104.441)
  line L8 (-19.5, 104.441) -> (-19.5, 65.441)
  line L9 (-19.5, 65.441) -> (19.5, 104.441) construction
  line L10 (19.5, 65.441) -> (-19.5, 104.441) construction
  circle A0 centre (0, 84.941) radius 12.5
  line L11 (-5, 73.4846) -> (-5, 69.941)
  line L12 (-5, 69.941) -> (5, 69.941)
  line L13 (5, 69.941) -> (5, 73.4846)
  point P0 (0, 84.941)
  dimension "d76" = 39
  dimension "d77" = 1.5
  dimension "d78" = 25
  dimension "d79" = 10
  dimension "d80" = 15
  constraint midpoint L0 L4.start
  constraint midpoint L2 L4.end
  constraint horizontal L5
  constraint perpendicular L5 L6
  constraint parallel L5 L7
  constraint parallel L6 L8
  constraint coincident L9 P0
  constraint coincident L10 P0
  constraint coincident L4 P0
  constraint equal L7 L8
  constraint coincident P0 A0.centre
  constraint coincident A0 L11.start
  constraint vertical L11
  constraint perpendicular L11 L12
  constraint coincident A0 L13.end
  constraint perpendicular L12 L13
  constraint symmetric L4 L11.end L12.end
  measures "d76" distance of L6.end L7.end
  measures "d77" distance of L0 L7
  measures "d78" diameter of A0
  measures "d79" distance of L11.end L12.end
  measures "d80" distance of P0 L12
extrude "拉伸4" cut sketch "草图10" against normal blind 3 contours L5 L6 L7 L8 | A0 | A0 L11 L12 L13
extrude "拉伸5" cut sketch "草图10" against normal up to surface (5 mm away) contours A0 | A0 L11 L12 L13
sketch "草图11" plane through (0, 17.4065, 6.3354) normal (0, 0.939693, 0.34202) x (-1, 0, 0)
  line L0 (5, 69.941) -> (-5, 69.941)
  line L1 (-5, 69.941) -> (-5, 73.4846)
  arc A0 (5, 73.4846) -> (-5, 73.4846) centre (0, 84.941) ccw
  line L2 (5, 73.4846) -> (5, 69.941)
  line L3 (-19.5, 104.441) -> (-19.5, 65.441)
  line L4 (-19.5, 65.441) -> (19.5, 65.441)
  line L5 (19.5, 65.441) -> (19.5, 104.441)
  line L6 (19.5, 104.441) -> (-19.5, 104.441)
  circle A1 centre (-14, 98.941) radius 0.9
  circle A2 centre (-14, 70.941) radius 0.9
  circle A3 centre (14, 70.941) radius 0.9
  circle A4 centre (14, 98.941) radius 0.9
  line L7 (0, 104.441) -> (0, 65.441) construction
  circle A5 centre (-14, 98.941) radius 2
  circle A6 centre (-14, 70.941) radius 2
  circle A7 centre (14, 70.941) radius 2
  circle A8 centre (14, 98.941) radius 2
  dimension "d81" = 1.8
  dimension "d83" = 360
  dimension "d84" = 28
  dimension "d85" = 4
  constraint midpoint L6 L7.start
  constraint midpoint L4 L7.end
  constraint symmetric A1.centre A4.centre L7
  constraint concentric A1 A5
  measures "d81" diameter of A1
  measures "d84" horizontal distance of A1.centre A4.centre
  measures "d85" diameter of A5
extrude "拉伸11" add sketch "草图11" along normal blind 2 contours A5 | A6 | A7 | A8
chamfer "倒角4" distance 2 angle 45 4 edges at (15.8647, -16.6807, 99.9892) (-12.1353, -16.6807, 99.9892) (-12.1353, -7.1041, 73.6778) (15.8647, -7.1041, 73.6778)
extrude "拉伸12" cut 4 faces at (14.4671, -16.4911, 99.4684) (-13.5329, -16.3755, 99.1508) (-13.5329, -6.9146, 73.157) (14.4671, -6.799, 72.8394) along direction (0, -0.939693, -0.34202) blind 2
chamfer "倒角5" distance 10 angle 45 2 edges at (-21, -3, 19.2678) (21, -3, 19.2678)
fillet "圆角2" radius 5 4 edges at (-13.0515, -3, 25.3359) (13.0515, -3, 25.3359) (-21, -3, 29.2678) (21, -3, 29.2678)
sketch "草图13" plane through (0, 0, 0) normal (0, 1, 0) x (-1, 0, 0)
  arc A0 (-21, 32.3728) -> (-18.217, 27.8911) centre (-16, 32.3728) ccw
  line L0 (-18.217, 27.8911) -> (-15.2017, 26.3995)
  arc A1 (-15.2017, 26.3995) -> (-11.0467, 26.2721) centre (-12.9847, 30.8812) ccw
  arc A2 (11.0467, 26.2721) -> (-11.0467, 26.2721) centre (0, 0) ccw
  arc A3 (11.0467, 26.2721) -> (15.2017, 26.3995) centre (12.9847, 30.8812) ccw
  line L1 (15.2017, 26.3995) -> (18.217, 27.8911)
  arc A4 (18.217, 27.8911) -> (21, 32.3728) centre (16, 32.3728) ccw
  line L2 (21, 32.3728) -> (21, 62.9308)
  line L3 (21, 62.9308) -> (-21, 62.9308)
  line L4 (-21, 62.9308) -> (-21, 32.3728)
  circle A5 centre (-10, 36) radius 1.8
  circle A6 centre (10, 36) radius 1.8
  circle A7 centre (16, 52.9308) radius 1.6
  circle A8 centre (16, 44.9308) radius 1.6
  dimension "d103" = 10
  dimension "d104" = 8
  dimension "d105" = 3.2
  dimension "d108" = 5
  constraint equal A7 A8
  constraint vertical A7.centre A8.centre
  measures "d103" distance of L3 A7.centre
  measures "d104" vertical distance of A7.centre A8.centre
  measures "d105" diameter of A7
  measures "d108" distance of L2 A7.centre
extrude "拉伸14" cut sketch "草图13" against normal blind 15 contours A7 | A8

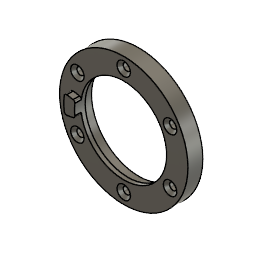
design "yaw轴承底座cnc版"
part number: 2026-07-22-14-30-40-374
Autodesk Fusion 360 part; units mm, degrees
sketch "草图1" plane through (0, 0, 0) normal (0, 0, 1) x (1, 0, 0)
  circle A0 centre (0, 0) radius 30
  circle A1 centre (0, 0) radius 22
  circle A2 centre (0, 0) radius 25 construction
  circle A3 centre (0, 25) radius 1.7
  circle A4 centre (-21.6506, 12.5) radius 1.7
  circle A5 centre (-21.6506, -12.5) radius 1.7
  circle A6 centre (0, -25) radius 1.7
  circle A7 centre (21.6506, -12.5) radius 1.7
  circle A8 centre (21.6506, 12.5) radius 1.7
  dimension "d1" = 60
  dimension "d2" = 44
  dimension "d3" = 50
  dimension "d4" = 3.4
  dimension "d6" = 360
  constraint coincident A0.centre A1.centre
  constraint concentric A1 A2
  constraint coincident A2 A3.centre
  measures "d1" diameter of A0
  measures "d2" diameter of A1
  measures "d3" diameter of A2
  measures "d4" diameter of A3
extrude "拉伸1" add sketch "草图1" along normal blind 5
sketch "草图2" plane through (0, 0, 5) normal (0, 0, 1) x (1, 0, 0)
  circle A0 centre (0, -25) radius 1.7
  circle A1 centre (21.6506, -12.5) radius 1.7
  circle A2 centre (-21.6506, 12.5) radius 1.7
  circle A3 centre (-21.6506, -12.5) radius 1.7
  circle A4 centre (21.6506, 12.5) radius 1.7
  circle A5 centre (0, 0) radius 22
  circle A6 centre (0, 25) radius 1.7
  circle A7 centre (0, 0) radius 30
  circle A8 centre (0, 0) radius 20
  dimension "d9" = 40
  constraint concentric A5 A8
  measures "d9" diameter of A8
extrude "拉伸2" add sketch "草图2" along normal blind 2 contours A5 | A7
hole "孔1" at (0, 25, 7) direction (0, 0, -1) diameter 3.3 depth 2 tip angle 180 countersink diameter 6.3 countersink angle 90
pattern_circular "C-阵列1" count 6 over 360 about axis through (0, 0, 1.75) along (0, 0, 1) of "孔1"
sketch "草图3" plane through (0, 0, 7) normal (0, 0, 1) x (1, 0, 0)
  circle A0 centre (21.6506, -12.5) radius 3.15
  circle A1 centre (-21.6506, -12.5) radius 3.15
  circle A2 centre (0, 25) radius 3.15
  circle A3 centre (0, 0) radius 20
  circle A4 centre (0, 0) radius 30
  circle A5 centre (-21.6506, 12.5) radius 3.15
  circle A6 centre (0, -25) radius 3.15
  circle A7 centre (21.6506, 12.5) radius 3.15
  line L0 (0, 0) -> (-24.6202, 4.3412)
  line L1 (0, 0) -> (-37, 0)
  line L2 (0, 0) -> (-24.6202, -4.3412)
  circle A8 centre (0, 0) radius 25
  dimension "d19" = 10
  dimension "d20" = 10
  dimension "d26" = 50
  constraint coincident A3.centre A4.centre
  constraint horizontal L1
  constraint coincident L0.end A8
  constraint coincident L2.end A8
  measures "d19" angle of L0 L1
  measures "d20" angle of L1 L2
  measures "d26" diameter of A8
extrude "拉伸3" add sketch "草图3" along normal blind 3 contours A3 L1 L2 A8 | A3 L0 L1 A8
fillet "圆角1" radius 1 4 edges at (-24.6202, 4.3412, 8.5) (-24.6202, -4.3412, 8.5) (-19.6962, -3.473, 8.5) (-19.6962, 3.473, 8.5)
sketch "草图6" plane through (0, 0, 0) normal (0, 0, -1) x (-1, 0, 0)
  circle A0 centre (-21.6506, 12.5) radius 1.7
  circle A1 centre (0, 25) radius 1.7
  circle A2 centre (-21.6506, -12.5) radius 1.7
  circle A3 centre (0, 0) radius 22
  circle A4 centre (0, -25) radius 1.7
  circle A5 centre (21.6506, 12.5) radius 1.7
  circle A6 centre (21.6506, -12.5) radius 1.7
  circle A7 centre (0, 0) radius 30
  circle A8 centre (0, 0) radius 37.5
  circle A9 centre (0, 0) radius 33.75
  circle A10 centre (-0.0757, -33.7499) radius 1.6
  circle A11 centre (16.8094, -29.2662) radius 1.6
  circle A12 centre (29.1904, -16.9405) radius 1.6
  circle A13 centre (33.7499, -0.0757) radius 1.6
  circle A14 centre (29.2662, 16.8094) radius 1.6
  circle A15 centre (16.9405, 29.1904) radius 1.6
  circle A16 centre (0.0757, 33.7499) radius 1.6
  circle A17 centre (-16.8094, 29.2662) radius 1.6
  circle A18 centre (-29.1904, 16.9405) radius 1.6
  circle A19 centre (-33.7499, 0.0757) radius 1.6
  circle A20 centre (-29.2662, -16.8094) radius 1.6
  circle A21 centre (-16.9405, -29.1904) radius 1.6
  dimension "d36" = 75
  dimension "d37" = 67.5
  dimension "d38" = 3.2
  dimension "d40" = 360
  constraint concentric A3 A8
  constraint concentric A8 A9
  constraint coincident A9 A10.centre
  measures "d36" diameter of A8
  measures "d37" diameter of A9
  measures "d38" diameter of A10

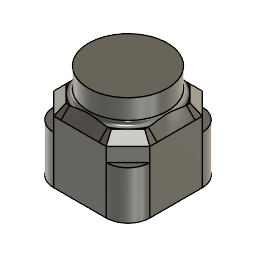
design "摄像头（防水）"
part number: 2026-07-20-15-06-44-368
Autodesk Fusion 360 part; units mm, degrees
sketch "草图1" plane through (0, 0, 0) normal (0, 0, 1) x (1, 0, 0)
  line L0 (0, 0) -> (22, 0)
  line L1 (22, 0) -> (22, 22)
  line L2 (22, 22) -> (0, 22)
  line L3 (0, 22) -> (0, 0)
  dimension "d1" = 22
  dimension "d2" = 22
  constraint horizontal L0
  constraint vertical L1
  constraint horizontal L2
  constraint vertical L3
  constraint coincident L0.start L3.end
  measures "d1" distance of L0.start L2.end
  measures "d2" distance of L1.end L2.end
extrude "拉伸1" add sketch "草图1" along normal blind 11
fillet "圆角3" radius 5 4 edges at (22, 0, 5.5) (0, 0, 5.5) (0, 22, 5.5) (22, 22, 5.5)
sketch "草图2" plane through (0, 0, 11) normal (0, 0, 1) x (-1, 0, 0)
  arc A0 (0, -5) -> (-5, 0) centre (-5, -5) ccw
  line L0 (-5, 0) -> (-17, 0)
  arc A1 (-17, 0) -> (-22, -5) centre (-17, -5) ccw
  line L1 (-22, -5) -> (-22, -17)
  line L2 (-17, -22) -> (-5, -22)
  line L3 (0, -17) -> (0, -5)
  line L4 (0, -17) -> (-5, -22)
  line L5 (-5, -22) -> (-17, -22)
  line L6 (-17, -22) -> (-22, -17)
  line L7 (-22, -17) -> (-22, -5)
  line L8 (-22, -5) -> (-17, 0)
  line L9 (-17, 0) -> (-5, 0)
  line L10 (-5, 0) -> (0, -5)
  line L11 (0, -17) -> (0, -5)
  arc A2 (-22, -17) -> (-17, -22) centre (-17, -17) ccw
  arc A3 (-5, -22) -> (0, -17) centre (-5, -17) ccw
  constraint coincident L3.start L4.start
  constraint coincident L2.end L4.end
  constraint coincident L2.start L5.end
  constraint coincident L1.end L6.end
  constraint coincident A1.end L1.start
  constraint coincident L0.end A1.start
  constraint coincident A0.end L0.start
  constraint coincident A0.start L3.end
extrude "拉伸2" add sketch "草图2" along normal blind 5.2 contours L0 L1 L2 L3 L4 L5 L6 L7 L8 L9 L10 L11